Autodesk Fusion 360 part; units mm, degrees
(part 2 of 2)
  constraint tangent L244 A250
  constraint tangent L245 A250
  constraint tangent L244 A251
  constraint tangent L248 A251
  constraint tangent L246 A252
  constraint tangent L247 A253
  constraint concentric A3 A254
  constraint concentric A4 A255
  constraint concentric A0 A256
  constraint concentric A1 A257
  constraint concentric A111 A258
  constraint concentric A112 A259
  constraint vertical L243
  constraint tangent L249 A260
  constraint tangent L250 A260
  constraint tangent L249 A261
  constraint tangent L243 A262
  constraint tangent L184 A263
  constraint tangent L185 A263
  constraint tangent L179 A264
  constraint tangent L180 A264
  constraint tangent L190 A265
  constraint tangent L189 A265
  constraint tangent L194 A266
  constraint tangent L195 A266
  constraint perpendicular L208 L251
  constraint coincident L208 L251.end
  constraint tangent L251 A267
  constraint tangent L250 A267
  constraint tangent A196 L252
  constraint tangent A253 L253
  constraint tangent L243 A268
  measures "d1" diameter of A0
  measures "d2" diameter of A1
  measures "d3" diameter of A2
  measures "d4" diameter of A3
  measures "d5" diameter of A4
  measures "d9" diameter of A111
  measures "d12" diameter of A112
  measures "d367" diameter of A254
  measures "d368" diameter of A255
  measures "d369" diameter of A256
  measures "d370" diameter of A257
  measures "d393" diameter of A258
  measures "d394" diameter of A259
extrude "Extrude1" add sketch "mriya-classic-fdm" along normal blind 10.6 contours L177 L178 L199 A206 L200 A207 L201 A208 L202 A209 L203 A210 L204 A211 L205 A212 L206 A213 L207 A214 L208 L209 A216 L210 A217 L211 A218 L212 A219 L213 A220 L214 A221 L215 A222 L216 A223 L217 A224 L218 A225 L219 A226 L220 A227 L221 L222 L223 L224 L225 L226 L227 L228 L229 L230 L231 L232 L233 L234 L235 L236 L237 L238 L239 L240 L241 L242 A228 A229 A231 A232 A233 A234 A235 A236 A237 A238 A239 A240 A241 A242 A243 A244 A245 A246 A247 A248 A249 makes body 1
extrude "Extrude2" add sketch "mriya-classic-fdm" along normal blind 17.1 contours L177 L178 L208 A215 L209 L236 L237 A230 bodies 1
extrude "Extrude3" add sketch "mriya-classic-fdm" along normal blind 3.7 contours A114 | A115 | A116 | A117 | L199 A206 L200 A207 L201 A208 L202 A209 L203 A210 L204 A211 L205 A212 L206 A213 L207 A214 L208 L209 A216 L210 A217 L211 A218 L212 A219 L213 A220 L214 A221 L215 A222 L216 A223 L217 A224 L218 A225 L219 A226 L220 A227 L243 L249 L250 A260 A261 A262 A267 A268 | L208 A215 L209 L249 L250 A260 A261 A267 | L208 L243 A262 A268 | A258 | A259 bodies 1
extrude "Extrude13" add sketch "mriya-classic-fdm" along normal blind 1.8 contours A2 | L108 L109 A118 A119 A120 L184 L185 A263 | A121 L110 A122 L111 A123 L179 L180 A264 | A124 L112 A125 L113 A126 L114 A127 L115 | A128 L116 A129 L117 A130 L118 A131 L119 | A132 L120 A133 A134 L121 L186 L187 L188 A198 A199 | A135 L122 A136 A137 L123 L181 L182 L183 A200 A201 | A138 L124 A139 L125 A140 L126 A141 L127 | A142 L128 A143 L129 A144 L130 A145 L131 | A146 L132 A147 L133 A148 L134 A149 L135 | A150 L136 A151 L137 A152 L138 A153 L139 | A154 L140 A155 L141 A156 L142 A157 L143 | A158 L144 A159 L145 A160 L146 A161 L147 | A162 L148 A163 L149 A164 L150 A165 L151 | A166 L152 A167 L153 A168 L191 L192 L193 A202 A203 | A169 L154 A170 L155 A171 L156 A172 L157 | A173 L158 A174 L159 A175 L196 L197 L198 A204 A205 | A176 L160 A177 L161 A178 L162 A179 L163 | A180 A181 L164 A182 L165 L194 L195 A266 | A183 L166 A184 L167 A185 L168 A186 L169 | A187 A188 L170 A189 L171 L189 L190 A265 | A190 L172 A191 L173 A192 L174 A193 L175 | A194 L176 A195 L244 L245 L248 A250 A251 | A196 A197 L246 L247 A252 A253 L252 L253 bodies 1
extrude "Extrude14" add sketch "mriya-classic-fdm" along normal blind 2.7 contours A0 | A1 | A3 | A4 bodies 1
extrude "Extrude6" add sketch "mriya-classic-fdm" along normal blind 1 from surface at 14.3 contours L208 A215 L209 L249 L250 A260 A261 A267 bodies 1
extrude "Extrude12" add sketch "mriya-classic-fdm" along normal blind 1 from surface at 7.7 contours L208 L243 A262 A268 bodies 1
sketch "power switch" plane through (-4.4, 0, 0) normal (1, 0, 0) x (0, 1, 0)
  line L0 (1.7932, 0) -> (76.6932, 0)
  line L1 (76.6932, 0) -> (76.6932, 17.1)
  line L2 (76.6932, 17.1) -> (19.2932, 17.1)
  line L3 (19.2932, 17.1) -> (19.2932, 10.6)
  line L4 (19.2932, 10.6) -> (1.7932, 10.6)
  line L5 (1.7932, 10.6) -> (1.7932, 0)
  line L6 (23.9932, 4.45) -> (23.9932, 9.3)
  line L7 (37.3932, 4.05) -> (24.3932, 4.05)
  arc A0 (37.7932, 9.3) -> (37.3932, 9.7) centre (37.3932, 9.3) ccw
  line L8 (36.0932, 8.35) -> (36.0932, 5.4)
  line L9 (25.6932, 8.35) -> (36.0932, 8.35)
  line L10 (36.0932, 5.4) -> (25.6932, 5.4)
  line L11 (25.6932, 5.4) -> (25.6932, 8.35)
  line L12 (24.3932, 9.7) -> (37.3932, 9.7)
  arc A1 (23.9932, 4.45) -> (24.3932, 4.05) centre (24.3932, 4.45) ccw
  arc A2 (37.3932, 4.05) -> (37.7932, 4.45) centre (37.3932, 4.45) ccw
  line L13 (37.7932, 9.3) -> (37.7932, 4.45)
  arc A3 (24.3932, 9.7) -> (23.9932, 9.3) centre (24.3932, 9.3) ccw
  constraint perpendicular L10 L11
  constraint vertical L11
  constraint perpendicular L9 L11
  constraint vertical L8
  constraint tangent A0 L12
  constraint tangent A0 L13
  constraint tangent A2 L13
  constraint tangent L7 A2
  constraint tangent L7 A1
  constraint tangent L6 A1
  constraint tangent L6 A3
  constraint tangent L12 A3
extrude "Extrude8" cut sketch "power switch" against normal blind 2.5 contours L8 L9 L10 L11 bodies 1
extrude "Extrude9" cut sketch "power switch" against normal blind 1 contours L6 L7 A0 L12 A1 A2 L13 A3 bodies 1
chamfer "Chamfer13" distance 1.19 angle 40 8 edges at (-4.4, 30.8932, 4.05) (-4.4, 24.1104, 4.1672) (-4.4, 23.9932, 6.875) (-4.4, 24.1104, 9.5828) (-4.4, 30.8932, 9.7) (-4.4, 37.676, 9.5828) (-4.4, 37.7932, 6.875) (-4.4, 37.676, 4.1672) measured on face at (-4.4, 63.7265, 8.8) measured on face at (-4.4, 63.7265, 8.8) measured on face at (-4.4, 63.7265, 8.8) measured on face at (-4.4, 63.7265, 8.8) measured on face at (-4.4, 63.7265, 8.8) measured on face at (-4.4, 63.7265, 8.8) measured on face at (-4.4, 63.7265, 8.8) measured on face at (-4.4, 63.7265, 8.8) on bodies 1
chamfer "Chamfer14" distance 0.5 angle 45 4 edges at (-6.9, 30.8932, 5.4) (-6.9, 25.6932, 6.875) (-6.9, 30.8932, 8.35) (-6.9, 36.0932, 6.875) on bodies 1
sketch "usb-c" plane through (0, 80.6932, 0) normal (0, 1, 0) x (-1, 0, 0)
  line L0 (8.4, 0) -> (41.0674, 0)
  line L1 (41.0674, 0) -> (41.0674, 10.6)
  line L2 (41.0674, 10.6) -> (25.8, 10.6)
  line L3 (25.8, 10.6) -> (25.8, 17.1)
  line L4 (25.8, 17.1) -> (8.4, 17.1)
  line L5 (8.4, 17.1) -> (8.4, 0)
  line L6 (19.7002, 8.8) -> (13.1003, 8.8)
  line L7 (21.8003, 12.8) -> (21.8003, 8.4)
  line L8 (21.0002, 11.1) -> (21.0002, 10.1)
  arc A0 (11.4003, 13.2) -> (11.0003, 12.8) centre (11.4003, 12.8) ccw
  arc A1 (21.4002, 8) -> (21.8002, 8.4) centre (21.4002, 8.4) ccw
  line L9 (11.8003, 10.1) -> (11.8003, 11.1)
  line L10 (21.4002, 8) -> (11.4002, 8)
  line L11 (11.4003, 13.2) -> (21.4002, 13.2)
  line L12 (13.1003, 12.4) -> (19.7002, 12.4)
  arc A2 (21.8002, 12.8) -> (21.4002, 13.2) centre (21.4002, 12.8) ccw
  arc A3 (11.0002, 8.4) -> (11.4002, 8) centre (11.4002, 8.4) ccw
  line L13 (11.0002, 8.4) -> (11.0003, 12.8)
  arc A4 (13.1003, 12.4) -> (11.8003, 11.1) centre (13.1003, 11.1) ccw
  arc A5 (11.8003, 10.1) -> (13.1003, 8.8) centre (13.1003, 10.1) ccw
  arc A6 (21.0002, 11.1) -> (19.7002, 12.4) centre (19.7002, 11.1) ccw
  arc A7 (19.7002, 8.8) -> (21.0002, 10.1) centre (19.7002, 10.1) ccw
  constraint perpendicular L7 L11
  constraint perpendicular L10 L13
  constraint horizontal L10
  constraint perpendicular L7 L10
  constraint tangent A0 L11
  constraint tangent A0 L13
  constraint tangent L11 A2
  constraint tangent L7 A2
  constraint tangent A3 L13
  constraint tangent L10 A3
  constraint tangent A1 L10
  constraint tangent L7 A1
  constraint tangent L12 A4
  constraint tangent L9 A4
  constraint tangent L9 A5
  constraint tangent L6 A5
  constraint tangent L8 A6
  constraint tangent L12 A6
  constraint tangent L6 A7
  constraint tangent L8 A7
extrude "Extrude17" cut sketch "usb-c" against normal blind 2.5 contours L6 L8 L9 L12 A4 A5 A6 A7 bodies 1
extrude "Extrude18" cut sketch "usb-c" against normal blind 1 contours L7 A0 A1 L10 L11 A2 A3 L13 bodies 1
chamfer "Chamfer23" distance 1.19 angle 40 8 edges at (-16.4003, 80.6932, 8) (-11.1174, 80.6932, 8.1172) (-11.0003, 80.6932, 10.6) (-11.1174, 80.6932, 13.0828) (-16.4003, 80.6932, 13.2) (-21.6831, 80.6932, 13.0828) (-21.8003, 80.6932, 10.6) (-21.6831, 80.6932, 8.1172) measured on face at (-23.6457, 80.6932, 2.6687) measured on face at (-23.6457, 80.6932, 2.6687) measured on face at (-23.6457, 80.6932, 2.6687) measured on face at (-23.6457, 80.6932, 2.6687) measured on face at (-23.6457, 80.6932, 2.6687) measured on face at (-23.6457, 80.6932, 2.6687) measured on face at (-23.6457, 80.6932, 2.6687) measured on face at (-23.6457, 80.6932, 2.6687) on bodies 1
chamfer "Chamfer21" distance 0.599 angle 45 3 edges at (-14.85, 78.1932, 14.3) (-7.3979, 77.6953, 14.3) (-6.9, 58.2432, 14.3) on bodies 1
chamfer "Chamfer22" distance 0.6 angle 45 1 edges at (-6.9, 9.5932, 7.7) on bodies 1
chamfer "Chamfer17" distance 1 angle 45 90 edges at (-17.0879, -2.2068, 10.6) (-5.5716, -1.0352, 10.6) (-4.4, 10.5432, 10.6) (-33.4337, 80.6932, 10.6) (-41.4501, 80.7693, 10.6) (-42.3387, 81.5503, 10.6) (-43.8762, 82.7648, 10.6) (-51.4458, 82.9932, 10.6) (-58.2501, 83.0693, 10.6) (-60.2387, 84.9503, 10.6) (-62.8762, 87.2648, 10.6) (-73.4, 87.4932, 10.6) (-83.9238, 87.2648, 10.6) (-86.0613, 85.4503, 10.6) (-87.5499, 84.0693, 10.6) (-94.8542, 83.9932, 10.6) (-102.9238, 83.7648, 10.6) (-107.238, 79.7735, 10.6) (-111.0657, 76.1074, 10.6) (-116.2077, 75.9932, 10.6) (-121.9238, 75.7648, 10.6) (-123.4613, 74.5503, 10.6) (-124.3499, 73.7693, 10.6) (-131.5163, 73.6932, 10.6) (-141.1284, 72.5216, 10.6) (-142.3, 42.8932, 10.6) (-141.1284, 13.2648, 10.6) (-120.4728, 12.0932, 10.6) (-100.9235, 12.4357, 10.6) (-96.4155, 16.4593, 10.6) (-92.7186, 19.941, 10.6) (-84.5898, 20.0932, 10.6) (-75.7143, 19.6842, 10.6) (-70.5474, 11.3702, 10.6) (-65.1972, 2.8703, 10.6) (-56.0828, 2.3932, 10.6) (-48.3499, 2.3171, 10.6) (-47.4613, 1.5361, 10.6) (-45.9238, 0.3216, 10.6) (-37.2542, 0.0932, 10.6) (-29.3499, 0.0171, 10.6) (-28.4613, -0.7639, 10.6) (-26.9238, -1.9784, 10.6) (-17.0879, -2.2068, 0) (-26.9238, -1.9784, 0) (-28.4613, -0.7639, 0) (-29.3499, 0.0171, 0) (-37.2542, 0.0932, 0) (-45.9238, 0.3216, 0) (-47.4613, 1.5361, 0) (-48.3499, 2.3171, 0) (-56.0828, 2.3932, 0) (-65.1972, 2.8703, 0) (-70.5474, 11.3702, 0) (-75.7143, 19.6842, 0) (-84.5898, 20.0932, 0) (-92.7186, 19.941, 0) (-96.4155, 16.4593, 0) (-100.9235, 12.4357, 0) (-120.4728, 12.0932, 0) (-141.1284, 13.2648, 0) (-142.3, 42.8932, 0) (-141.1284, 72.5216, 0) (-131.5163, 73.6932, 0) (-124.3499, 73.7693, 0) (-123.4613, 74.5503, 0) (-121.9238, 75.7648, 0) (-116.2077, 75.9932, 0) (-111.0657, 76.1074, 0) (-107.238, 79.7735, 0) (-102.9238, 83.7648, 0) (-94.8542, 83.9932, 0) (-87.5499, 84.0693, 0) (-86.0613, 85.4503, 0) (-83.9238, 87.2648, 0) (-73.4, 87.4932, 0) (-62.8762, 87.2648, 0) (-60.2387, 84.9503, 0) (-58.2501, 83.0693, 0) (-51.4458, 82.9932, 0) (-43.8762, 82.7648, 0) (-42.3387, 81.5503, 0) (-41.4501, 80.7693, 0) (-24.7337, 80.6932, 0) (-5.5716, 79.5216, 0) (-4.4, 39.2432, 0) (-5.5716, -1.0352, 0) (-4.4, 47.9932, 17.1) (-5.5716, 79.5216, 17.1) (-17.1, 80.6932, 17.1) on bodies 1
fillet "Fillet29" radius 1.2 2 edges at (-4.4, 19.2932, 12.85) (-25.8, 80.6932, 12.85) on bodies 1
chamfer "Chamfer18" distance 1 angle 45 4 edges at (-6.25, 19.2932, 17.1) (-5.4996, 19.2974, 17.1) (-25.8, 78.8432, 17.1) (-25.7958, 79.5936, 17.1) on bodies 1
chamfer "Chamfer20" distance 1 angle 45 6 edges at (-11.1722, 22.9091, 0) (-23.6722, 22.9091, 0) (-45.9722, 22.9591, 0) (-45.9722, 60.9591, 0) (-121.9722, 34.9591, 0) (-121.9722, 53.9591, 0) on bodies 1
sketch "silicone feets" plane through (0, 0, 0) normal (0, 0, -1) x (1, 0, 0)
  circle A0 centre (-120.9, -34.5432) radius 2.15
  circle A1 centre (-44.9, -22.5432) radius 2.15
  circle A2 centre (-10.1, -22.4932) radius 2.15
  line L0 (-8.4, 1.2068) -> (-25.7757, 1.2068)
  arc A3 (-25.7757, 1.2068) -> (-27.1899, 0.621) centre (-25.7757, -0.7932) ccw
  line L1 (-27.1899, 0.621) -> (-28.3184, -0.5074)
  arc A4 (-29.7326, -1.0932) -> (-28.3184, -0.5074) centre (-29.7326, 0.9068) ccw
  line L2 (-29.7326, -1.0932) -> (-44.7757, -1.0932)
  arc A5 (-44.7757, -1.0932) -> (-46.1899, -1.679) centre (-44.7757, -3.0932) ccw
  line L3 (-46.1899, -1.679) -> (-47.3184, -2.8074)
  arc A6 (-48.7326, -3.3932) -> (-47.3184, -2.8074) centre (-48.7326, -1.3932) ccw
  line L4 (-48.7326, -3.3932) -> (-63.4331, -3.3932)
  arc A7 (-63.4331, -3.3932) -> (-65.6097, -4.6635) centre (-63.4331, -5.8932) ccw
  line L5 (-65.6097, -4.6635) -> (-73.7438, -19.0608)
  arc A8 (-77.2264, -21.0932) -> (-73.7438, -19.0608) centre (-77.2264, -17.0932) ccw
  line L6 (-77.2264, -21.0932) -> (-91.9532, -21.0932)
  arc A9 (-94.0745, -20.2145) -> (-91.9532, -21.0932) centre (-91.9532, -18.0932) ccw
  line L7 (-94.0745, -20.2145) -> (-100.1707, -14.1183)
  arc A10 (-100.1707, -14.1183) -> (-102.6456, -13.0932) centre (-102.6456, -16.5932) ccw
  line L8 (-102.6456, -13.0932) -> (-138.3, -13.0932)
  arc A11 (-138.3, -13.0932) -> (-141.3, -16.0932) centre (-138.3, -16.0932) ccw
  line L9 (-141.3, -16.0932) -> (-141.3, -69.6932)
  arc A12 (-141.3, -69.6932) -> (-138.3, -72.6932) centre (-138.3, -69.6932) ccw
  line L10 (-138.3, -72.6932) -> (-124.7326, -72.6932)
  arc A13 (-123.3184, -73.279) -> (-124.7326, -72.6932) centre (-124.7326, -74.6932) ccw
  line L11 (-123.3184, -73.279) -> (-122.1899, -74.4074)
  arc A14 (-122.1899, -74.4074) -> (-120.7757, -74.9932) centre (-120.7757, -72.9932) ccw
  line L12 (-120.7757, -74.9932) -> (-111.6397, -74.9932)
  arc A15 (-109.8719, -75.7254) -> (-111.6397, -74.9932) centre (-111.6397, -77.4932) ccw
  line L13 (-109.8719, -75.7254) -> (-103.19, -82.4074)
  arc A16 (-103.19, -82.4074) -> (-101.7757, -82.9932) centre (-101.7757, -80.9932) ccw
  line L14 (-101.7757, -82.9932) -> (-87.9326, -82.9932)
  arc A17 (-86.5184, -83.579) -> (-87.9326, -82.9932) centre (-87.9326, -84.9932) ccw
  line L15 (-86.5184, -83.579) -> (-84.19, -85.9074)
  arc A18 (-84.19, -85.9074) -> (-82.7757, -86.4932) centre (-82.7757, -84.4932) ccw
  line L16 (-82.7757, -86.4932) -> (-64.0243, -86.4932)
  arc A19 (-64.0243, -86.4932) -> (-62.6101, -85.9074) centre (-64.0243, -84.4932) ccw
  line L17 (-62.6101, -85.9074) -> (-59.2816, -82.579)
  arc A20 (-57.8674, -81.9932) -> (-59.2816, -82.579) centre (-57.8674, -83.9932) ccw
  line L18 (-57.8674, -81.9932) -> (-45.0243, -81.9932)
  arc A21 (-45.0243, -81.9932) -> (-43.6101, -81.4074) centre (-45.0243, -79.9932) ccw
  line L19 (-43.6101, -81.4074) -> (-42.4816, -80.279)
  arc A22 (-41.0674, -79.6932) -> (-42.4816, -80.279) centre (-41.0674, -81.6932) ccw
  line L20 (-41.0674, -79.6932) -> (-8.4, -79.6932)
  arc A23 (-8.4, -79.6932) -> (-5.4, -76.6932) centre (-8.4, -76.6932) ccw
  line L21 (-5.4, -76.6932) -> (-5.4, -1.7932)
  arc A24 (-5.4, -1.7932) -> (-8.4, 1.2068) centre (-8.4, -1.7932) ccw
  circle A25 centre (-22.6, -22.4932) radius 2.15
  circle A26 centre (-44.9, -60.5432) radius 2.15
  circle A27 centre (-120.9, -53.5432) radius 2.15
  circle A28 centre (-11.9, -73.1932) radius 4.1
  circle A29 centre (-73.4, -79.9932) radius 4.1
  circle A30 centre (-134.8, -66.1932) radius 4.1
  circle A31 centre (-134.8, -19.5932) radius 4.1
  circle A32 centre (-61.0987, -9.8932) radius 4.1
  circle A33 centre (-11.9, -5.2932) radius 4.1
  dimension "d374" = 8.2
  dimension "d375" = 8.2
  dimension "d376" = 8.2
  dimension "d377" = 8.2
  dimension "d378" = 8.2
  dimension "d379" = 8.2
  dimension "d380" = 6.5
  dimension "d381" = 6.5
  dimension "d382" = 6.5
  dimension "d383" = 6.5
  dimension "d384" = 6.5
  dimension "d385" = 6.5
  dimension "d386" = 6.5
  dimension "d387" = 6.5
  dimension "d388" = 6.5
  dimension "d389" = 6.5
  dimension "d390" = 6.5
  measures "d374" diameter of A28
  measures "d375" diameter of A29
  measures "d376" diameter of A30
  measures "d377" diameter of A31
  measures "d378" diameter of A32
  measures "d379" diameter of A33
  measures "d380" distance of L20 A28.centre
  measures "d381" distance of L21 A28.centre
  measures "d382" distance of L16 A29.centre
  measures "d383" distance of L10 A30.centre
  measures "d384" distance of L9 A30.centre
  measures "d385" distance of L9 A31.centre
  measures "d386" distance of L8 A31.centre
  measures "d387" distance of L5 A32.centre
  measures "d388" distance of L4 A32.centre
  measures "d389" distance of L0 A33.centre
  measures "d390" distance of L21 A33.centre
extrude "Extrude15" cut sketch "silicone feets" against normal blind 0.9 contours A28 | A29 | A30 | A31 | A32 | A33 bodies 1
extrude "Extrude16" cut sketch "mriya-classic-fdm" along normal blind 1 from surface at 2.7 contours A258 | A259 bodies 1
mirror "Mirror1" about plane through (0, 0, 0) normal (1, 0, 0) of bodies 1 makes body 2
named bodies: "Left", "Right"
